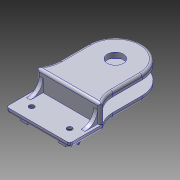
# Autodesk Inventor part: CableHolder
Saved by Autodesk Inventor 2013 (Build 170138000, 138)
## iProperties
Created: 2013-11-09
Part Number: CableHolder
Material: Generic
Document SubType Name: Modeling
Designer: JustinIndra
Density: 1 g/cm^3
Author: JustinIndra
Autodesk Inventor part; units mm, degrees
ref_plane "YZ Plane" through (0, 0, 0) normal (1, 0, 0) x (0, 1, 0)
ref_plane "XZ Plane" through (0, 0, 0) normal (0, 1, 0) x (-1, 0, 0)
ref_plane "XY Plane" through (0, 0, 0) normal (0, 0, 1) x (1, 0, 0)
sketch "Sketch1" plane through (0, 0, 0) normal (0, 1, 0) x (-1, 0, 0)
  line L0 (10.5, -28) -> (-10.5, -28)
  line L1 (-10.5, -28) -> (-10.5, 0)
  line L2 (-10.5, 0) -> (10.5, 0)
  line L3 (10.5, 0) -> (10.5, -28)
  circle A0 centre (0, -17.5) radius 3.175
  point P0 (0, 0)
  point P1 (0, 0)
  dimension "d0" = 21
  dimension "d2" = 17.5
  dimension "d3" = 6.35
  dimension "d4" = 10.5
  constraints: 8 end point, 2 coincident, 2 parallel, 1 centre point, 1 horizontal, 1 midpoint, 1 perpendicular, 1 vertical alignment
  measures "d0" distance of L0.start L0.end
  measures "d2" distance from line of L2 A0.centre
  measures "d3" diameter of A0
  measures "d4" distance from line of A0.centre L0
extrude "Extrusion1" add sketch "Sketch1" along normal mid plane 9.35
sketch "Sketch2" plane through (-10.5, 4.675, 0) normal (0, 0, 1) x (1, 0, 0)
  line L0 (0, 0) -> (21, 0) projected
  line L1 (21, -9.35) -> (0, -9.35) projected
  line L2 (-2, 0) -> (23, 0)
  line L3 (23, 0) -> (23, -9.35)
  line L4 (23, -9.35) -> (-2, -9.35)
  line L5 (-2, -9.35) -> (-2, 0)
  point P0 (10.5, -4.675)
  point P1 (10.5, 0)
  dimension "d10" = 25
  constraints: 8 end point, 2 collinear, 2 parallel, 1 horizontal, 1 midpoint, 1 perpendicular, 1 vertical alignment
  measures "d10" distance of L3.end L4.end
sketch "Sketch3" plane through (10.5, 4.675, -28) normal (0, 0, -1) x (-1, 0, 0)
  line L0 (21, -9.35) -> (21, 0) projected
  line L1 (0, 0) -> (0, -9.35) projected
  line L2 (21, -9.35) -> (0, -9.35) projected
  line L3 (0, -2) -> (21, -2)
  line L4 (21, -2) -> (21, -7.35)
  line L5 (21, -7.35) -> (0, -7.35)
  line L6 (0, -7.35) -> (0, -2)
  point P0 (10.5, -4.675)
  point P1 (0, -4.675)
  dimension "d7" = 2
  constraints: 8 end point, 2 parallel, 2 point on line, 1 horizontal, 1 horizontal alignment, 1 midpoint, 1 perpendicular
  measures "d7" distance between parallel lines of L2 L5
extrude "Extrusion2" cut sketch "Sketch3" against normal up to next contours L5 L1 L3 L0
extrude "Extrusion3" add sketch "Sketch2" along normal blind 1
sketch "Sketch4" plane through (-10.5, 4.675, 1) normal (0, 0, 1) x (1, 0, 0)
  line L0 (-2, 0) -> (-2, -9.35) projected
  line L1 (-2, -7.35) -> (23, -7.35)
  line L2 (23, -7.35) -> (23, -9.35)
  line L3 (23, -9.35) -> (-2, -9.35)
  line L4 (-2, -9.35) -> (-2, -7.35)
  point P0 (10.5, -4.675)
  dimension "d14" = 2
  constraints: 8 end point, 2 parallel, 1 horizontal, 1 perpendicular, 1 point on line
  measures "d14" distance of L3.end L1.start
extrude "Extrusion4" add sketch "Sketch4" along normal blind 12
sketch "Sketch6" plane through (0, -4.675, 0) normal (0, -1, 0) x (1, 0, 0)
  line L0 (-12.5, 13) -> (12.5, 13) projected
  line L1 (-12.5, 0) -> (-12.5, 13) projected
  line L2 (-4.6132, 8) -> (-6.0566, 5.5)
  line L3 (-6.0566, 5.5) -> (-8.9434, 5.5)
  line L4 (-8.9434, 5.5) -> (-10.3868, 8)
  line L5 (-10.3868, 8) -> (-8.9434, 10.5)
  line L6 (-8.9434, 10.5) -> (-6.0566, 10.5)
  line L7 (-6.0566, 10.5) -> (-4.6132, 8)
  point P0 (0, 0)
  point P1 (-7.5, 8)
  point P2 (-7.5, 8)
  dimension "d18" = 5
  dimension "d19" = 5
  dimension "d20" = 5
  constraints: 12 end point, 1 coincident, 1 horizontal, 13 other
  measures "d18" distance between parallel lines of L3 L6
  measures "d19" distance from line of L0 point (-7.5, 8)
  measures "d20" distance from line of L1 point (-7.5, 8)
hole "Hole1" at (-7.5, -4.675, 8) direction (0, 1, 0) diameter 2.013 end through all thread size "M2.5x0.45" class "6H" standard "ISO Metric profile"
extrude "Extrusion5" cut sketch "Sketch6" against normal blind 1
sketch "Sketch7" plane through (0, -4.675, 0) normal (0, -1, 0) x (1, 0, 0)
  line L0 (-4.6132, 8) -> (-6.0566, 5.5) projected
  line L1 (-8.9434, 5.5) -> (-10.3868, 8) projected
  line L2 (-8.9434, 10.5) -> (-6.0566, 10.5) projected
  line L3 (-8.9434, 11) -> (-6.0566, 11)
  line L4 (-6.0566, 11) -> (-6.0566, 10.5)
  line L5 (-6.0566, 10.5) -> (-8.9434, 10.5)
  line L6 (-8.9434, 10.5) -> (-8.9434, 11)
  line L7 (-4.6132, 8) -> (-6.0566, 5.5)
  line L8 (-6.0566, 5.5) -> (-5.6236, 5.25)
  line L9 (-5.6236, 5.25) -> (-4.1802, 7.75)
  line L10 (-4.1802, 7.75) -> (-4.6132, 8)
  line L11 (-8.9434, 5.5) -> (-10.3868, 8)
  line L12 (-10.3868, 8) -> (-10.8198, 7.75)
  line L13 (-10.8198, 7.75) -> (-9.3764, 5.25)
  line L14 (-9.3764, 5.25) -> (-8.9434, 5.5)
  point P0 (0, 0)
  dimension "d30" = 0.5
  constraints: 24 end point, 9 equal length, 3 perpendicular, 1 horizontal, 1 point on line
  measures "d30" distance of L3.end L2.end
extrude "Extrusion6" add sketch "Sketch7" along normal blind 1
sketch "Sketch8" plane through (0, -5.675, 0) normal (0, -1, 0) x (1, 0, 0)
  line L0 (-6.0566, 11) -> (-8.9434, 11) projected
  line L1 (-8.9434, 10.5) -> (-6.0566, 10.5) projected
  line L2 (-10.8198, 7.75) -> (-9.5207, 8.5)
  line L3 (-9.5207, 8.5) -> (-8.0774, 6)
  line L4 (-8.0774, 6) -> (-9.3764, 5.25)
  line L5 (-9.3764, 5.25) -> (-10.8198, 7.75)
  line L6 (-5.4793, 8.5) -> (-4.1802, 7.75)
  line L7 (-4.1802, 7.75) -> (-5.6236, 5.25)
  line L8 (-5.6236, 5.25) -> (-6.9226, 6)
  line L9 (-6.9226, 6) -> (-5.4793, 8.5)
  line L10 (-8.9434, 11) -> (-6.0566, 11)
  line L11 (-6.0566, 11) -> (-6.0566, 9.5)
  line L12 (-6.0566, 9.5) -> (-8.9434, 9.5)
  line L13 (-8.9434, 9.5) -> (-8.9434, 11)
  line L14 (-10.8198, 7.75) -> (-9.3764, 5.25) projected
  line L15 (-9.3764, 5.25) -> (-8.9434, 5.5) projected
  line L16 (-10.3868, 8) -> (-10.8198, 7.75) projected
  line L17 (-6.0566, 5.5) -> (-5.6236, 5.25) projected
  line L18 (-5.6236, 5.25) -> (-4.1802, 7.75) projected
  line L19 (-4.1802, 7.75) -> (-4.6132, 8) projected
  point P0 (0, 0)
  dimension "d33" = 1
  constraints: 24 end point, 9 equal length, 6 collinear, 3 perpendicular
  measures "d33" distance between parallel lines of L12 L1
extrude "Extrusion7" add sketch "Sketch8" along normal blind 1
chamfer "Chamfer1" distance 1 angle 45 3 edges at (-7.5, -6.675, 9.5) (-6.201, -6.675, 7.25) (-8.799, -6.675, 7.25)
mirror "Mirror1" about plane through (0, 0, 0) normal (1, 0, 0) of "Hole1", "Extrusion5", "Extrusion6", "Extrusion7", "Chamfer1"
fillet "Fillet1" radius 10.5 4 edges at (-10.5, 3.675, -28) (10.5, 3.675, -28) (-10.5, -3.675, -28) (10.5, -3.675, -28)
fillet "Fillet2" radius 10 4 edges at (-10.5, 3.675, 0) (-10.5, -3.675, 0) (10.5, -3.675, 0) (10.5, 3.675, 0)
fillet "Fillet3" radius 5 1 edges at (0, -2.675, 1)
sketch "Sketch9" plane through (-12.5, -2.675, 13) normal (0, 1, 0) x (1, 0, 0)
  line L0 (0, 7) -> (25, 7) projected
  line L1 (0, 7) -> (0, 0) projected
  line L2 (25, 0) -> (0, 0) projected
  circle A0 centre (5, 5) radius 1.0065 projected
  circle A1 centre (20, 5) radius 1.0065 projected
  line L3 (2.5, 0) -> (22.5, 0)
  line L4 (22.5, 0) -> (22.5, 12)
  line L5 (22.5, 12) -> (2.5, 12)
  line L6 (2.5, 12) -> (2.5, 0)
  line L7 (25, 12) -> (0, 12) projected
  line L8 (0, 0) -> (1, 0)
  line L9 (1, 0) -> (1, 12)
  line L10 (1, 12) -> (0, 12)
  line L11 (0, 12) -> (0, 0)
  line L12 (25, 0) -> (24, 0)
  line L13 (24, 0) -> (24, 12)
  line L14 (24, 12) -> (25, 12)
  line L15 (25, 12) -> (25, 0)
  point P0 (12.5, 13)
  point P1 (12.5, 0)
  point P2 (12.5, 7)
  dimension "d43" = 1.5
  dimension "d45" = 1
  constraints: 24 end point, 6 parallel, 3 horizontal, 3 perpendicular, 2 collinear, 2 equal length, 2 midpoint, 1 point on line, 1 vertical alignment
  measures "d43" distance between parallel lines of L6 L9
  measures "d45" distance between parallel lines of L1 L9
extrude "Extrusion8" cut sketch "Sketch9" along normal through all contours L11 L7 L9 L0 | L0 L9 L2 L1 | L6 L5 L4 L0 | L0 L4 L2 L6 | L13 L7 L15 L0 | L0 L15 L2 L13
fillet "Fillet4" radius 1 28 edges at (12.5, -3.675, 13) (-12.5, -3.675, 13) (12.5, -4.675, 6.5) (0, -4.675, 13) (-12.5, -4.675, 6.5) (-12.5, 1, 1) (12.5, 1, 1) (-11.0132, 4.675, -2.8377) (7.4247, 4.675, -24.9247) (0, 4.675, -28) (-7.4247, 4.675, -24.9247) (10.5, 4.675, -11.7501) (11.0132, 4.675, -2.8377) (-10.5, 4.675, -11.7501) (7.4247, -4.675, -24.9247) (0, -4.675, -28) (-7.4247, -4.675, -24.9247) (10.5, -4.675, -11.7501) (11.0132, -4.675, -2.8377) (-11.0132, -4.675, -2.8377) (-10.5, -4.675, -11.7501) (-9.665, -6.675, 6.7501) (-7.5, -6.675, 10.4999) (-5.335, -6.675, 6.75) (7.5, -6.675, 10.4999) (5.335, -6.675, 6.75) (9.665, -6.675, 6.7501) (0, 4.675, 1)
equation "\"d4\" = 0.5 * d0"
body "Solid1"
